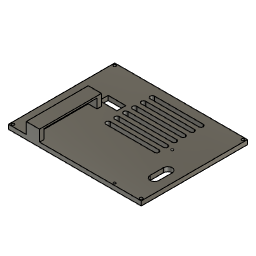
蓋 (Autodesk Fusion 360 design; units mm, degrees)
Autodesk Fusion 360 part; units mm, degrees
sketch "スケッチ1" plane through (0, 0, 0) normal (0, 0, 1) x (1, 0, 0)
  line L0 (75, -45) -> (-75, -45)
  line L1 (-75, -45) -> (-75, 75)
  line L2 (-75, 75) -> (75, 75)
  line L3 (75, 75) -> (75, -45)
  line L4 (-115.7726, 0) -> (130, 0)
  dimension "d1" = 150
  dimension "d41" = 75
  dimension "d42" = 45
  constraint horizontal L0
  constraint perpendicular L0 L1
  constraint parallel L0 L2
  constraint parallel L1 L3
  constraint horizontal L4
  measures "d1" distance of L1.end L2.end
  measures "d41" distance of L2 L4
  measures "d42" distance of L0 L4
extrude "押し出し1" add sketch "スケッチ1" along normal blind 5
sketch "スケッチ2" plane through (0, 0, 5) normal (0, 0, 1) x (-1, 0, 0)
  line L0 (-75, -75) -> (75, -75)
  line L1 (75, -75) -> (75, 45)
  line L2 (75, 45) -> (-75, 45)
  line L3 (-75, 45) -> (-75, -75)
  circle A0 centre (72.5, -72.5) radius 1.5
  line L4 (0, -100) -> (0, -20)
  circle A1 centre (-72.5, -72.5) radius 1.5
  line L5 (50, 0) -> (-80, 0)
  circle A2 centre (72.5, 72.5) radius 1.5
  circle A3 centre (-72.5, 72.5) radius 1.5
  dimension "d5" = 3
  dimension "d6" = 2.5
  dimension "d7" = 2.5
  constraint vertical L4
  constraint symmetric A0 L4 A1
  constraint perpendicular L3 L5
  constraint symmetric A0 L5 A2
  constraint symmetric A1 L5 A3
  measures "d5" diameter of A0
  measures "d6" distance of L0 A0.centre
  measures "d7" distance of L1 A0.centre
extrude "押し出し2" cut sketch "スケッチ2" against normal blind 5 contours A0 | A1 | A2 | A3
sketch "スケッチ3" plane through (0, 0, 5) normal (0, 0, 1) x (-1, 0, 0)
  circle A0 centre (-72.5, -72.5) radius 1.5
  circle A1 centre (72.5, -72.5) radius 1.5
  line L0 (-75, -75) -> (75, -75)
  line L1 (75, -75) -> (75, 45)
  line L2 (75, 45) -> (-75, 45)
  line L3 (-75, 45) -> (-75, -75)
  line L4 (47, -39.5) -> (27, -39.5)
  line L5 (27, -39.5) -> (27, -29.5)
  line L6 (27, -29.5) -> (47, -29.5)
  line L7 (47, -29.5) -> (47, -39.5)
  dimension "d10" = 28
  dimension "d11" = 45.5
  dimension "d12" = 10
  dimension "d13" = 20
  constraint horizontal L4
  constraint vertical L5
  constraint horizontal L6
  constraint vertical L7
  measures "d10" distance of L1 L7
  measures "d11" distance of L0 L6
  measures "d12" distance of L4 L6
  measures "d13" distance of L5 L7
extrude "押し出し3" cut sketch "スケッチ3" against normal blind 5 contours L4 L5 L6 L7
sketch "スケッチ4" plane through (0, 0, 5) normal (0, 0, 1) x (-1, 0, 0)
  line L0 (27, -39.5) -> (27, -29.5)
  line L1 (27, -29.5) -> (47, -29.5)
  line L2 (47, -29.5) -> (47, -39.5)
  line L3 (47, -39.5) -> (27, -39.5)
  circle A0 centre (-72.5, -72.5) radius 1.5
  circle A1 centre (72.5, -72.5) radius 1.5
  line L4 (-75, -75) -> (75, -75)
  line L5 (75, -75) -> (75, 45)
  line L6 (75, 45) -> (-75, 45)
  line L7 (-75, 45) -> (-75, -75)
  line L8 (20, -65) -> (-35, -65)
  line L9 (-35, -60) -> (20, -60)
  line L10 (20, -55) -> (-35, -55)
  line L11 (-35, -50) -> (20, -50)
  line L12 (20, -45) -> (-35, -45)
  line L13 (-35, -40) -> (20, -40)
  line L14 (20, -35) -> (-35, -35)
  line L15 (-35, -30) -> (20, -30)
  line L16 (20, -25) -> (-35, -25)
  line L17 (-35, -20) -> (20, -20)
  line L18 (20, -15) -> (-35, -15)
  line L19 (-35, -10) -> (20, -10)
  arc A2 (20, -65) -> (20, -60) centre (20, -62.5) ccw
  arc A3 (20, -55) -> (20, -50) centre (20, -52.5) ccw
  arc A4 (20, -45) -> (20, -40) centre (20, -42.5) ccw
  arc A5 (20, -35) -> (20, -30) centre (20, -32.5) ccw
  arc A6 (20, -25) -> (20, -20) centre (20, -22.5) ccw
  arc A7 (20, -15) -> (20, -10) centre (20, -12.5) ccw
  arc A8 (-35, -10) -> (-35, -15) centre (-35, -12.5) ccw
  arc A9 (-35, -20) -> (-35, -25) centre (-35, -22.5) ccw
  arc A10 (-35, -30) -> (-35, -35) centre (-35, -32.5) ccw
  arc A11 (-35, -40) -> (-35, -45) centre (-35, -42.5) ccw
  arc A12 (-35, -50) -> (-35, -55) centre (-35, -52.5) ccw
  arc A13 (-35, -60) -> (-35, -65) centre (-35, -62.5) ccw
  constraint horizontal L8
  constraint horizontal L9
  constraint horizontal L10
  constraint horizontal L11
  constraint horizontal L12
  constraint horizontal L13
  constraint horizontal L14
  constraint horizontal L15
  constraint horizontal L16
  constraint horizontal L17
  constraint horizontal L18
  constraint horizontal L19
  constraint tangent L8 A2
  constraint tangent L10 A3
  constraint tangent L12 A4
  constraint tangent L14 A5
  constraint tangent L16 A6
  constraint tangent L18 A7
  constraint tangent L19 A8
  constraint tangent L17 A9
  constraint tangent L15 A10
  constraint tangent L13 A11
  constraint tangent L11 A12
  constraint tangent L9 A13
extrude "押し出し4" cut sketch "スケッチ4" against normal blind 5 contours L8 L9 A2 A13 | L10 L11 A3 A12 | L12 L13 A4 A11 | L14 L15 A5 A10 | L16 L17 A6 A9 | L18 L19 A7 A8
sketch "スケッチ5" plane through (0, 0, 5) normal (0, 0, 1) x (-1, 0, 0)
  line L0 (-35, -30) -> (20, -30)
  arc A0 (20, -35) -> (20, -30) centre (20, -32.5) ccw
  line L1 (20, -35) -> (-35, -35)
  arc A1 (-35, -30) -> (-35, -35) centre (-35, -32.5) ccw
  line L2 (-35, -60) -> (20, -60)
  arc A2 (20, -65) -> (20, -60) centre (20, -62.5) ccw
  line L3 (20, -65) -> (-35, -65)
  arc A3 (-35, -60) -> (-35, -65) centre (-35, -62.5) ccw
  line L4 (-35, -50) -> (20, -50)
  arc A4 (20, -55) -> (20, -50) centre (20, -52.5) ccw
  line L5 (20, -55) -> (-35, -55)
  arc A5 (-35, -50) -> (-35, -55) centre (-35, -52.5) ccw
  line L6 (-35, -20) -> (20, -20)
  arc A6 (20, -25) -> (20, -20) centre (20, -22.5) ccw
  line L7 (20, -25) -> (-35, -25)
  arc A7 (-35, -20) -> (-35, -25) centre (-35, -22.5) ccw
  line L8 (-35, -10) -> (20, -10)
  arc A8 (20, -15) -> (20, -10) centre (20, -12.5) ccw
  line L9 (20, -15) -> (-35, -15)
  arc A9 (-35, -10) -> (-35, -15) centre (-35, -12.5) ccw
  line L10 (-35, -40) -> (20, -40)
  arc A10 (20, -45) -> (20, -40) centre (20, -42.5) ccw
  line L11 (20, -45) -> (-35, -45)
  arc A11 (-35, -40) -> (-35, -45) centre (-35, -42.5) ccw
  line L12 (27, -39.5) -> (27, -29.5)
  line L13 (27, -29.5) -> (47, -29.5)
  line L14 (47, -29.5) -> (47, -39.5)
  line L15 (47, -39.5) -> (27, -39.5)
  circle A12 centre (-72.5, -72.5) radius 1.5
  circle A13 centre (72.5, -72.5) radius 1.5
  line L16 (-75, -75) -> (75, -75)
  line L17 (75, -75) -> (75, 45)
  line L18 (75, 45) -> (-75, 45)
  line L19 (-75, 45) -> (-75, -75)
  line L20 (50, -20) -> (40, -20)
  line L21 (40, 40) -> (50, 40)
  line L22 (50, 40) -> (50, -20)
  line L23 (55, -25) -> (40, -25)
  line L24 (40, 45) -> (55, 45)
  line L25 (55, 45) -> (55, -25)
  line L26 (40, -25) -> (40, -20)
  line L27 (40, 40) -> (40, 45)
  circle A14 centre (-52.5, -22.5) radius 1.5
  circle A15 centre (-52.5, 42.5) radius 1.5
  dimension "d18" = 60
  dimension "d20" = 3
  dimension "d21" = 3
  dimension "d22" = 2.5
  dimension "d25" = 2.5
  constraint horizontal L20
  constraint horizontal L21
  constraint vertical L22
  constraint horizontal L23
  constraint horizontal L24
  constraint vertical L25
  constraint perpendicular L21 L26
  constraint collinear L26 L27
  measures "d18" distance of L20 L21
  measures "d20" diameter of A14
  measures "d21" diameter of A15
  measures "d22" distance of L23 A14.centre
  measures "d25" distance of L24 A15.centre
extrude "押し出し5" add sketch "スケッチ5" along normal blind 10.7 contours L18 L20 L21 L22 L23 L24 L25 L26 L27
sketch "スケッチ7" plane through (0, 0, 15.7) normal (0, 0, 1) x (-1, 0, 0)
  line L0 (50, 40) -> (50, -20)
  line L1 (50, -20) -> (40, -20)
  line L2 (40, -20) -> (40, -25)
  line L3 (40, -25) -> (55, -25)
  line L4 (55, -25) -> (55, 45)
  line L5 (55, 45) -> (40, 45)
  line L6 (40, 45) -> (40, 40)
  line L7 (40, 40) -> (50, 40)
  line L8 (55, -25) -> (40, -25)
  line L9 (40, -25) -> (40, 45)
  line L10 (40, 45) -> (55, 45)
  line L11 (55, 45) -> (55, -25)
  constraint horizontal L8
  constraint vertical L9
  constraint horizontal L10
  constraint vertical L11
  constraint coincident L5.end L6.start
  constraint coincident L3.end L4.start
extrude "押し出し6" add sketch "スケッチ7" along normal blind 2
sketch "スケッチ8" plane through (0, 0, 5) normal (0, 0, 1) x (-1, 0, 0)
  line L0 (50, 40) -> (40, 40)
  line L1 (40, 40) -> (40, 45)
  line L2 (40, 45) -> (-75, 45)
  line L3 (55, 45) -> (55, -25)
  line L4 (55, -25) -> (40, -25)
  line L5 (40, -25) -> (40, -20)
  line L6 (40, -20) -> (50, -20)
  line L7 (50, -20) -> (50, 40)
  line L8 (-35, -30) -> (20, -30)
  arc A0 (20, -35) -> (20, -30) centre (20, -32.5) ccw
  line L9 (20, -35) -> (-35, -35)
  arc A1 (-35, -30) -> (-35, -35) centre (-35, -32.5) ccw
  line L10 (-35, -60) -> (20, -60)
  arc A2 (20, -65) -> (20, -60) centre (20, -62.5) ccw
  line L11 (20, -65) -> (-35, -65)
  arc A3 (-35, -60) -> (-35, -65) centre (-35, -62.5) ccw
  line L12 (-35, -50) -> (20, -50)
  arc A4 (20, -55) -> (20, -50) centre (20, -52.5) ccw
  line L13 (20, -55) -> (-35, -55)
  arc A5 (-35, -50) -> (-35, -55) centre (-35, -52.5) ccw
  line L14 (-35, -20) -> (20, -20)
  arc A6 (20, -25) -> (20, -20) centre (20, -22.5) ccw
  line L15 (20, -25) -> (-35, -25)
  arc A7 (-35, -20) -> (-35, -25) centre (-35, -22.5) ccw
  line L16 (-35, -10) -> (20, -10)
  arc A8 (20, -15) -> (20, -10) centre (20, -12.5) ccw
  line L17 (20, -15) -> (-35, -15)
  arc A9 (-35, -10) -> (-35, -15) centre (-35, -12.5) ccw
  line L18 (-35, -40) -> (20, -40)
  arc A10 (20, -45) -> (20, -40) centre (20, -42.5) ccw
  line L19 (20, -45) -> (-35, -45)
  arc A11 (-35, -40) -> (-35, -45) centre (-35, -42.5) ccw
  line L20 (27, -39.5) -> (27, -29.5)
  line L21 (27, -29.5) -> (47, -29.5)
  line L22 (47, -29.5) -> (47, -39.5)
  line L23 (47, -39.5) -> (27, -39.5)
  circle A12 centre (-72.5, -72.5) radius 1.5
  circle A13 centre (72.5, -72.5) radius 1.5
  line L24 (-75, -75) -> (75, -75)
  line L25 (75, -75) -> (75, 45)
  line L26 (75, 45) -> (55, 45)
  line L27 (-75, 45) -> (-75, -75)
  line L28 (55, -25) -> (-45, -25)
  line L29 (-45, -25) -> (-45, 45)
  line L30 (-45, 45) -> (55, 45)
  line L31 (55, 45) -> (55, -25)
  circle A14 centre (-42.5, -22.5) radius 1.5
  circle A15 centre (-42.5, 42.5) radius 1.5
  dimension "d30" = 3
  dimension "d31" = 2.5
  dimension "d32" = 2.5
  dimension "d33" = 3
  dimension "d34" = 2.5
  dimension "d35" = 2.5
  constraint horizontal L28
  constraint vertical L29
  constraint horizontal L30
  constraint vertical L31
  constraint coincident L3.end L4.start
  measures "d30" diameter of A14
  measures "d31" distance of L28 A14.centre
  measures "d32" distance of L29 A14.centre
  measures "d33" diameter of A15
  measures "d34" distance of L29 A15.centre
  measures "d35" distance of L30 A15.centre
hole "穴1" at (42.5, 22.5, 5) at (42.5, -42.5, 5) direction (0, 0, -1) diameter 2.529 depth 10 tip angle 118
thread "ねじ1" "ISO Metric profile 3.0 M3x0.5 6H"
sketch "スケッチ9" plane through (0, 0, 5) normal (0, 0, 1) x (-1, 0, 0)
  circle A0 centre (-42.5, -22.5) radius 1.2645
  circle A1 centre (-42.5, 42.5) radius 1.2645
  line L0 (50, 40) -> (40, 40)
  line L1 (40, 40) -> (40, 45)
  line L2 (40, 45) -> (-75, 45)
  line L3 (55, 45) -> (55, -25)
  line L4 (55, -25) -> (40, -25)
  line L5 (40, -25) -> (40, -20)
  line L6 (40, -20) -> (50, -20)
  line L7 (50, -20) -> (50, 40)
  line L8 (-35, -30) -> (20, -30)
  arc A2 (20, -35) -> (20, -30) centre (20, -32.5) ccw
  line L9 (20, -35) -> (-35, -35)
  arc A3 (-35, -30) -> (-35, -35) centre (-35, -32.5) ccw
  line L10 (-35, -60) -> (20, -60)
  arc A4 (20, -65) -> (20, -60) centre (20, -62.5) ccw
  line L11 (20, -65) -> (-35, -65)
  arc A5 (-35, -60) -> (-35, -65) centre (-35, -62.5) ccw
  line L12 (-35, -50) -> (20, -50)
  arc A6 (20, -55) -> (20, -50) centre (20, -52.5) ccw
  line L13 (20, -55) -> (-35, -55)
  arc A7 (-35, -50) -> (-35, -55) centre (-35, -52.5) ccw
  line L14 (-35, -20) -> (20, -20)
  arc A8 (20, -25) -> (20, -20) centre (20, -22.5) ccw
  line L15 (20, -25) -> (-35, -25)
  arc A9 (-35, -20) -> (-35, -25) centre (-35, -22.5) ccw
  line L16 (-35, -10) -> (20, -10)
  arc A10 (20, -15) -> (20, -10) centre (20, -12.5) ccw
  line L17 (20, -15) -> (-35, -15)
  arc A11 (-35, -10) -> (-35, -15) centre (-35, -12.5) ccw
  line L18 (-35, -40) -> (20, -40)
  arc A12 (20, -45) -> (20, -40) centre (20, -42.5) ccw
  line L19 (20, -45) -> (-35, -45)
  arc A13 (-35, -40) -> (-35, -45) centre (-35, -42.5) ccw
  line L20 (27, -39.5) -> (27, -29.5)
  line L21 (27, -29.5) -> (47, -29.5)
  line L22 (47, -29.5) -> (47, -39.5)
  line L23 (47, -39.5) -> (27, -39.5)
  circle A14 centre (-72.5, -72.5) radius 1.5
  circle A15 centre (72.5, -72.5) radius 1.5
  line L24 (-75, -75) -> (75, -75)
  line L25 (75, -75) -> (75, 45)
  line L26 (75, 45) -> (55, 45)
  line L27 (-75, 45) -> (-75, -75)
  line L28 (-65, 0) -> (-65, 15)
  line L29 (-55, 15) -> (-55, 0)
  arc A16 (-65, 0) -> (-55, 0) centre (-60, 0) ccw
  arc A17 (-55, 15) -> (-65, 15) centre (-60, 15) ccw
  constraint vertical L28
  constraint vertical L29
  constraint tangent L29 A16
  constraint tangent L29 A17
extrude "押し出し7" cut sketch "スケッチ9" against normal blind 5 contours L28 L29 A16 A17
sketch "スケッチ10" plane through (0, 0, 5) normal (0, 0, 1) x (-1, 0, 0)
  line L0 (-55, 15) -> (-55, 0)
  arc A0 (-65, 0) -> (-55, 0) centre (-60, 0) ccw
  line L1 (-65, 0) -> (-65, 15)
  arc A1 (-55, 15) -> (-65, 15) centre (-60, 15) ccw
  circle A2 centre (-42.5, -22.5) radius 1.2645
  circle A3 centre (-42.5, 42.5) radius 1.2645
  line L2 (55, 45) -> (55, -25)
  line L3 (55, -25) -> (40, -25)
  line L4 (40, -25) -> (40, -20)
  line L5 (40, -20) -> (50, -20)
  line L6 (50, -20) -> (50, 40)
  line L7 (50, 40) -> (40, 40)
  line L8 (40, 40) -> (40, 45)
  line L9 (40, 45) -> (-75, 45)
  line L10 (-75, 45) -> (-75, -75)
  line L11 (-75, -75) -> (75, -75)
  line L12 (75, -75) -> (75, 45)
  line L13 (75, 45) -> (55, 45)
  circle A4 centre (72.5, -72.5) radius 1.5
  circle A5 centre (-72.5, -72.5) radius 1.5
  line L14 (27, -39.5) -> (27, -29.5)
  line L15 (27, -29.5) -> (47, -29.5)
  line L16 (47, -29.5) -> (47, -39.5)
  line L17 (47, -39.5) -> (27, -39.5)
  line L18 (-35, -40) -> (20, -40)
  arc A6 (20, -45) -> (20, -40) centre (20, -42.5) ccw
  line L19 (20, -45) -> (-35, -45)
  arc A7 (-35, -40) -> (-35, -45) centre (-35, -42.5) ccw
  line L20 (-35, -10) -> (20, -10)
  arc A8 (20, -15) -> (20, -10) centre (20, -12.5) ccw
  line L21 (20, -15) -> (-35, -15)
  arc A9 (-35, -10) -> (-35, -15) centre (-35, -12.5) ccw
  line L22 (-35, -20) -> (20, -20)
  arc A10 (20, -25) -> (20, -20) centre (20, -22.5) ccw
  line L23 (20, -25) -> (-35, -25)
  arc A11 (-35, -20) -> (-35, -25) centre (-35, -22.5) ccw
  line L24 (-35, -50) -> (20, -50)
  arc A12 (20, -55) -> (20, -50) centre (20, -52.5) ccw
  line L25 (20, -55) -> (-35, -55)
  arc A13 (-35, -50) -> (-35, -55) centre (-35, -52.5) ccw
  line L26 (-35, -60) -> (20, -60)
  arc A14 (20, -65) -> (20, -60) centre (20, -62.5) ccw
  line L27 (20, -65) -> (-35, -65)
  arc A15 (-35, -60) -> (-35, -65) centre (-35, -62.5) ccw
  line L28 (-35, -30) -> (20, -30)
  arc A16 (20, -35) -> (20, -30) centre (20, -32.5) ccw
  line L29 (20, -35) -> (-35, -35)
  arc A17 (-35, -30) -> (-35, -35) centre (-35, -32.5) ccw
  circle A18 centre (72.5, 42.5) radius 1.5
  circle A19 centre (-72.5, 42.5) radius 1.5
  dimension "d43" = 3
  dimension "d44" = 2.5
  dimension "d45" = 2.5
  dimension "d46" = 3
  dimension "d47" = 2.5
  dimension "d48" = 2.5
  measures "d43" diameter of A18
  measures "d44" distance of L12 A18.centre
  measures "d45" distance of L13 A18.centre
  measures "d46" diameter of A19
  measures "d47" distance of L10 A19.centre
  measures "d48" distance of L9 A19.centre
extrude "押し出し8" cut sketch "スケッチ10" against normal blind 5 contours A18 | A19
equation "d11 = 35 mm + 10.50 mm"
equation "d42 = 75 mm - 30 mm"
